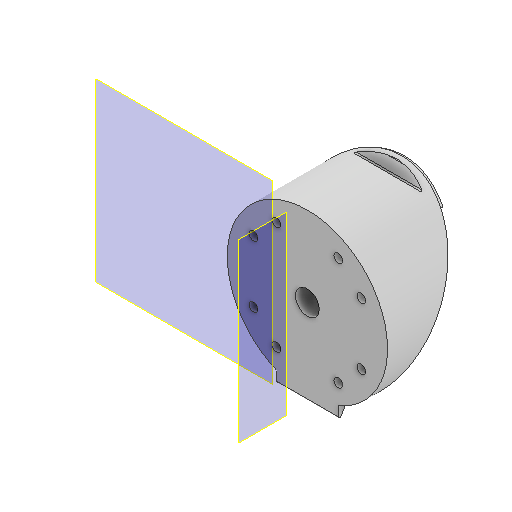
# Autodesk Inventor part: Spectrometer_gratingholder_v0
Saved by Autodesk Inventor 2022 (Build 260153000, 153)
## iProperties
Created: 2022-03-20
Part Number: Spectrometer_gratingholder_v0
Material: Generic
Document SubType Name: Modeling
Designer: Prakash Lab
Density: 1 g/cm^3
Appearance: Default
Author: Prakash Lab
Autodesk Inventor part; units mm, degrees
ref_plane "YZ Plane" through (0, 0, 0) normal (1, 0, 0) x (0, 1, 0)
ref_plane "XZ Plane" through (0, 0, 0) normal (0, 1, 0) x (-1, 0, 0)
ref_plane "Work Plane1" through (-54.6514, -58.9369, 28.8009) normal (0, 0, -1) x (-1, 0, 0)
ref_plane "Arbeitsebene5" through (-88.1514, -83.8908, 20.4259) normal (0, 0.5, 0.8660254) x (1, 0, 0)
sketch "Sketch1" plane through (-50.6514, -58.9369, 28.8009) normal (0, 0, 1) x (1, 0, 0)
  circle A0 centre (-11.9999, -12.4979) radius 25.9979 projected
  circle A1 centre (-2, 4.9999) radius 1.3999 projected
  circle A2 centre (-22, 5) radius 1.4 projected
  circle A3 centre (-12, -12.5) radius 3.85 projected
  line L0 (-5, -5) -> (-5, 0) projected
  line L1 (0, 0) -> (0, -5) projected
  circle A4 centre (-22, -30) radius 1.4 projected
  circle A5 centre (-2, -30) radius 1.4001 projected
  line L2 (-5, 0) -> (0, 0)
  line L3 (0, 0) -> (0, -5)
  line L4 (0, -5) -> (-5, -5)
  line L5 (-5, -5) -> (-5, 0)
  circle A6 centre (-12, -12.5) radius 4
  point P0 (50.6514, 58.9369)
  dimension "d2" = 8
  constraints: 8 end point, 2 parallel, 1 centre point, 1 coincident, 1 horizontal, 1 perpendicular, 1 other
  measures "d2" diameter of A6
extrude "Extrusion1" add sketch "Sketch1" against normal up to surface contours A0 | L0 L2 L1 L4 | A6 surface through (-88.1514, -83.8908, 20.4259) normal (0, 0.5, 0.8660254)
sketch "Skizze17" plane through (-62.6512, -71.4348, 13.2343) normal (0, -0.5, -0.8660254) x (-1, 0, 0)
  line L0 (23.5002, 23.867) -> (-23.4998, 23.867) projected
  arc A0 (-23.4998, 23.867) -> (-25.4998, 21.867) centre (-23.4998, 21.867) ccw projected
  line L1 (-25.4998, 21.867) -> (-25.4998, -25.133) projected
  arc A1 (-25.4998, -25.133) -> (-23.4998, -27.133) centre (-23.4998, -25.133) ccw projected
  line L2 (-23.4998, -27.133) -> (23.5002, -27.133) projected
  arc A2 (23.5002, -27.133) -> (25.5002, -25.133) centre (23.5002, -25.133) ccw projected
  line L3 (25.5002, -25.133) -> (25.5002, 21.867) projected
  arc A3 (25.5002, 21.867) -> (23.5002, 23.867) centre (23.5002, 21.867) ccw projected
  line L4 (-17.4998, 11.367) -> (17.5002, 11.367) projected
  line L5 (17.5002, 11.367) -> (17.5002, -12.633) projected
  line L6 (17.5002, -12.633) -> (-17.4998, -12.633) projected
  line L7 (-17.4998, -12.633) -> (-17.4998, 11.367) projected
  line L8 (-23.4998, 24.067) -> (23.5002, 24.067)
  arc A4 (25.7002, 21.867) -> (23.5002, 24.067) centre (23.5002, 21.867) ccw
  line L9 (25.7002, 21.867) -> (25.7002, -25.133)
  arc A5 (23.5002, -27.333) -> (25.7002, -25.133) centre (23.5002, -25.133) ccw
  line L10 (23.5002, -27.333) -> (-23.4998, -27.333)
  arc A6 (-25.6998, -25.133) -> (-23.4998, -27.333) centre (-23.4998, -25.133) ccw
  line L11 (-25.6998, -25.133) -> (-25.6998, 21.867)
  arc A7 (-23.4998, 24.067) -> (-25.6998, 21.867) centre (-23.4998, 21.867) ccw
  ellipse E0 centre (-9.9998, 20.2048) end of major axis (-9.9998, 21.8213) minor radius 1.3999 projected
  ellipse E1 centre (10.0001, 20.2048) end of major axis (10.0001, 21.8213) minor radius 1.4 projected
  ellipse E2 centre (0.0001, -0.0025) end of major axis (0.0001, 4.4432) minor radius 3.85 projected
  ellipse E3 centre (10.0001, -20.2097) end of major axis (10.0001, -18.5931) minor radius 1.4 projected
  ellipse E4 centre (-9.9999, -20.2096) end of major axis (-9.9999, -18.593) minor radius 1.4001 projected
  ellipse E5 centre (0, 0) end of major axis (0, -30.0198) minor radius 25.9979 projected
  point P0 (-62.6512, 68.4815)
  point P1 (15.5395, 24.067)
  point P2 (-15.5395, 24.067)
  point P3 (10.7503, -27.333)
  point P4 (-10.7503, -27.333)
  dimension "d65" = 0.2
  constraints: 8 end point, 8 point on circle, 4 centre point, 8 other
  measures "d65" distance between parallel lines of L0 L8
extrude "Extrusion13" add sketch "Skizze17" along normal blind 1 contours L8 E5 | E5 L10
ref_plane "Arbeitsebene6" through (-62.6514, -59.1868, 48.3009) normal (-1, 0, 0) x (0, 0, -1)
sketch "Skizze18" plane through (-62.6514, -59.1868, 48.3009) normal (-1, 0, 0) x (0, 0, -1)
  line L0 (47.1, -8.5947) -> (47.1, -8.5947) projected
  line L1 (47.1, -8.5947) -> (47.966, -8.0947) projected
  line L2 (47.966, -8.0947) -> (47.966, -8.0947) projected
  line L3 (47.1, -8.5947) -> (47.966, -8.0947) projected
  line L4 (21.4, 35.919) -> (21.4, 35.919) projected
  line L5 (21.4, 35.919) -> (22.266, 36.419) projected
  line L6 (22.266, 36.419) -> (22.266, 36.419) projected
  line L7 (21.4, 35.919) -> (22.266, 36.419) projected
  line L8 (21.4, 35.919) -> (22.266, 36.419) projected
  line L9 (22.266, 36.419) -> (19.5, 34.8221)
  line L10 (19.5, 38.2458) -> (19.5, -13.75) projected
  line L11 (22.266, 36.419) -> (19.5, 34.8221)
  line L12 (22.266, 36.419) -> (20.9226, 38.7458) projected
  line L13 (22.266, 36.419) -> (20.433, 39.5939)
  line L14 (19.5, 39.3439) -> (19.5, 34.8221)
  arc A0 (20.433, 39.5939) -> (19.5, 39.3439) centre (20, 39.3439) ccw
  point P0 (48.3009, -59.1868)
  point P1 (19.5, 38.2458)
  point P2 (20.9226, 38.7458)
  dimension "d68" = 0.5
  constraints: 8 end point, 2 collinear, 2 point on circle, 2 tangent, 1 centre point, 1 point on line, 1 vertical
  measures "d68" radius of A0
extrude "Extrusion14" add sketch "Skizze18" along normal mid plane 20
sketch "Skizze19" plane through (-62.6514, -59.1868, 48.3009) normal (-1, 0, 0) x (0, 0, -1)
  line L0 (47.1, -8.5947) -> (47.1, -8.5947) projected
  line L1 (47.1, -8.5947) -> (47.966, -8.0947) projected
  line L2 (47.966, -8.0947) -> (47.966, -8.0947) projected
  line L3 (47.1, -8.5947) -> (47.966, -8.0947) projected
  line L4 (48.1255, -13.6035) -> (46.0052, -11.4832)
  line L5 (48.4791, -13.75) -> (51.4776, -13.75) construction
  line L6 (45.2981, -11.4832) -> (43.0314, -13.75)
  line L7 (19.5, -13.75) -> (50.0764, -13.75) projected
  line L8 (43.0314, -13.75) -> (48.272, -13.75)
  arc A0 (46.0052, -11.4832) -> (45.2981, -11.4832) centre (45.6517, -11.8368) ccw
  arc A1 (48.1255, -13.6035) -> (48.4791, -13.75) centre (48.4791, -13.25) ccw
  point P0 (48.3009, -59.1868)
  point P1 (48.4791, -13.75)
  dimension "d71" = 135
  dimension "d72" = 90
  dimension "d73" = 0.5
  constraints: 8 end point, 4 point on circle, 4 tangent, 3 point on line, 2 centre point, 1 collinear, 1 equal length, 1 equal radius, 1 horizontal
  measures "d71" angle of L5 L4
  measures "d72" angle of L6 L4
  measures "d73" radius of A0
extrude "Extrusion15" cut sketch "Skizze19" along normal through all both and the other way through all
sketch "Skizze20" plane through (-50.6514, -58.9369, 28.8009) normal (0, 0, 1) x (1, 0, 0)
  circle A0 centre (-29.4977, -2.4981) radius 1.3999
  circle A1 centre (-29.4977, -22.498) radius 1.4
  circle A2 centre (-11.9977, -12.498) radius 3.85
  circle A3 centre (5.5022, -22.498) radius 1.4
  circle A4 centre (5.5022, -2.498) radius 1.4001
  arc A5 (-2.0001, -36.4957) -> (-22.0001, -36.4955) centre (-11.9999, -12.4979) ccw
  line L0 (-22.0001, -39.5939) -> (-22.0001, -36.4955)
  line L1 (-22.0001, -39.5939) -> (-2.0001, -39.5939)
  line L2 (-2.0001, -36.4957) -> (-2.0001, -39.5939)
  line L3 (5.498, -22.4977) -> (5.498, -2.4981)
  line L4 (5.498, -2.4981) -> (-29.4977, -2.4981)
  line L5 (-29.4977, -2.4981) -> (-29.4977, -22.4977)
  line L6 (-29.4977, -22.4977) -> (5.498, -22.4977)
  line L7 (5.498, -22.4977) -> (-29.4977, -2.4981) construction
  line L8 (5.498, -2.4981) -> (-29.4977, -22.4977) construction
  point P0 (50.6514, 58.9369)
  constraints: 18 end point, 10 centre point, 2 midpoint, 2 parallel, 2 point on circle, 1 coincident with centre, 1 perpendicular
hole "Bohrung3" at (-80.1491, -61.4349, 28.8009) at (-80.1491, -81.4346, 28.8009) at (-45.1491, -81.4349, 28.8009) at (-45.1534, -61.4349, 28.8009) direction (0, 0, -1) diameter 2.8 depth 14 tip angle 118
body "Solid1"
